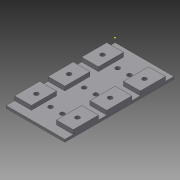
# Autodesk Inventor part: parking lot frame
Saved by Autodesk Inventor 2015 (Build 190159000, 159)
## iProperties
Created: 2015-10-07
Part Number: parking lot frame
Material: Generic
Document SubType Name: Modeling
Designer: Jason
Density: 1 g/cm^3
Appearance: Default
Author: Jason
Autodesk Inventor part; units mm, degrees
ref_plane "YZ Plane" through (0, 0, 0) normal (1, 0, 0) x (0, 1, 0)
ref_plane "XZ Plane" through (0, 0, 0) normal (0, 1, 0) x (-1, 0, 0)
ref_plane "XY Plane" through (0, 0, 0) normal (0, 0, 1) x (1, 0, 0)
sketch "Sketch1" plane through (0, 0, 0) normal (0, 0, 1) x (1, 0, 0)
  line L0 (0, 0) -> (70, 0)
  line L1 (70, 0) -> (70, -130)
  line L2 (70, -130) -> (0, -130)
  line L3 (0, -130) -> (0, 0)
  line L4 (0, -10) -> (20, -10)
  line L5 (20, -10) -> (20, -40)
  line L6 (20, -40) -> (0, -40)
  line L7 (0, -40) -> (0, -10)
  line L8 (50, -10) -> (70, -10)
  line L9 (70, -10) -> (70, -40)
  line L10 (70, -40) -> (50, -40)
  line L11 (50, -40) -> (50, -10)
  line L12 (0, -50) -> (20, -50)
  line L13 (20, -50) -> (20, -80)
  line L14 (20, -80) -> (0, -80)
  line L15 (0, -80) -> (0, -50)
  line L16 (50, -50) -> (70, -50)
  line L17 (70, -50) -> (70, -80)
  line L18 (70, -80) -> (50, -80)
  line L19 (50, -80) -> (50, -50)
  line L20 (0, -90) -> (20, -90)
  line L21 (20, -90) -> (20, -120)
  line L22 (20, -120) -> (0, -120)
  line L23 (0, -120) -> (0, -90)
  line L24 (50, -90) -> (70, -90)
  line L25 (70, -90) -> (70, -120)
  line L26 (70, -120) -> (50, -120)
  line L27 (50, -120) -> (50, -90)
  dimension "d0" = 70
  dimension "d1" = 130
  dimension "d2" = 20
  dimension "d3" = 30
  dimension "d4" = 20
  dimension "d5" = 30
  dimension "d6" = 20
  dimension "d7" = 30
  dimension "d8" = 20
  dimension "d9" = 30
  dimension "d10" = 20
  dimension "d11" = 30
  dimension "d12" = 20
  dimension "d13" = 30
  dimension "d14" = 10
  dimension "d15" = 10
  dimension "d16" = 10
  dimension "d17" = 10
  dimension "d18" = 10
  dimension "d19" = 0
  dimension "d20" = 30
  constraints: 56 end point, 14 parallel, 7 horizontal, 7 perpendicular, 5 point on line
  measures "d0" distance of L1.end L2.end
  measures "d1" distance between parallel lines of L2 L0
  measures "d2" distance of L5.end L6.end
  measures "d3" distance of L4.end L5.end
  measures "d4" distance of L9.end L10.end
  measures "d5" distance of L8.end L9.end
  measures "d6" distance of L13.end L14.end
  measures "d7" distance of L12.end L13.end
  measures "d8" distance of L17.end L18.end
  measures "d9" distance of L16.end L17.end
  measures "d10" distance of L21.end L22.end
  measures "d11" distance of L20.end L21.end
  measures "d12" distance of L25.end L26.end
  measures "d13" distance of L24.end L25.end
  measures "d14" distance between parallel lines of L0 L4
  measures "d15" distance between parallel lines of L12 L6
  measures "d16" distance between parallel lines of L20 L14
  measures "d17" distance between parallel lines of L16 L10
  measures "d18" distance between parallel lines of L24 L18
  measures "d19" distance between parallel lines of L23 L3
  measures "d20" distance between parallel lines of L27 L21
extrude "Extrusion1" add sketch "Sketch1" along normal blind 3 contours L0 L1 L8 L11 L10 L16 L19 L18 L24 L27 L26 L2 L3 L22 L21 L20 L14 L13 L12 L6 L5 L4
sketch "Sketch6" plane through (0, 0, 0) normal (0, 0, -1) x (-1, 0, 0)
  line L0 (-50, -10) -> (-70, -10)
  line L1 (-70, -10) -> (-70, -40)
  line L2 (-70, -40) -> (-50, -40)
  line L3 (-50, -40) -> (-50, -10)
  line L4 (-20, -10) -> (0, -10)
  line L5 (0, -10) -> (0, -40)
  line L6 (0, -40) -> (-20, -40)
  line L7 (-20, -40) -> (-20, -10)
  line L8 (-20, -50) -> (0, -50)
  line L9 (0, -50) -> (0, -80)
  line L10 (0, -80) -> (-20, -80)
  line L11 (-20, -80) -> (-20, -50)
  line L12 (0, -90) -> (-20, -90)
  line L13 (-20, -90) -> (-20, -120)
  line L14 (-20, -120) -> (0, -120)
  line L15 (0, -120) -> (0, -90)
  line L16 (-50, -90) -> (-70, -90)
  line L17 (-70, -90) -> (-70, -120)
  line L18 (-70, -120) -> (-50, -120)
  line L19 (-50, -120) -> (-50, -90)
  line L20 (-70, -80) -> (-50, -80)
  line L21 (-50, -80) -> (-50, -50)
  line L22 (-50, -50) -> (-70, -50)
  line L23 (-70, -50) -> (-70, -80)
  point P0 (0, 0)
  constraints: 48 end point, 12 parallel, 6 horizontal, 6 perpendicular
extrude "Extrusion3" add sketch "Sketch6" against normal blind 8
sketch "Sketch7" plane through (0, 0, 8) normal (0, 0, 1) x (1, 0, 0)
  point P0 (0, 0)
sketch "Sketch8" plane through (0, 0, 8) normal (0, 0, 1) x (1, 0, 0)
  circle A0 centre (10, -25) radius 2.6
  circle A1 centre (28, -25) radius 2.6
  circle A2 centre (42, -25) radius 2.6
  circle A3 centre (60, -25) radius 2.6
  circle A4 centre (10, -65) radius 2.6
  circle A5 centre (28, -65) radius 2.6
  circle A6 centre (42, -65) radius 2.6
  circle A7 centre (59, -65) radius 2.6
  circle A8 centre (11, -105) radius 2.6
  circle A9 centre (28, -105) radius 2.6
  circle A10 centre (42, -105) radius 2.6
  circle A11 centre (60, -105) radius 2.6
  line L0 (20, -10) -> (0, -10) projected
  line L1 (20, -40) -> (20, -10) projected
  line L2 (50, -10) -> (50, -40) projected
  line L3 (70, -10) -> (50, -10) projected
  line L4 (70, -40) -> (70, -10) projected
  line L5 (20, -50) -> (0, -50) projected
  line L6 (20, -90) -> (0, -90) projected
  line L7 (50, -50) -> (50, -80) projected
  point P0 (0, 0)
  dimension "d29" = 5.2
  dimension "d30" = 5.2
  dimension "d31" = 5.2
  dimension "d32" = 5.2
  dimension "d33" = 5.2
  dimension "d34" = 5.2
  dimension "d35" = 5.2
  dimension "d36" = 5.2
  dimension "d37" = 5.2
  dimension "d38" = 5.2
  dimension "d39" = 5.2
  dimension "d40" = 5.2
  dimension "d41" = 15
  dimension "d42" = 10
  dimension "d43" = 8
  dimension "d44" = 8
  dimension "d45" = 15
  dimension "d46" = 10
  dimension "d47" = 15
  dimension "d48" = 15
  dimension "d49" = 8
  constraints: 12 centre point
  measures "d29" diameter of A0
  measures "d30" diameter of A1
  measures "d31" diameter of A2
  measures "d32" diameter of A3
  measures "d33" diameter of A4
  measures "d34" diameter of A5
  measures "d35" diameter of A6
  measures "d36" diameter of A7
  measures "d37" diameter of A8
  measures "d38" diameter of A9
  measures "d39" diameter of A10
  measures "d40" diameter of A11
  measures "d41" distance from line of L0 A0.centre
  measures "d42" distance from line of L1 A0.centre
  measures "d43" distance from line of A1.centre L1
  measures "d44" distance from line of L2 A2.centre
  measures "d45" distance from line of L3 A3.centre
  measures "d46" distance from line of L4 A3.centre
  measures "d47" distance from line of L5 A4.centre
  measures "d48" distance from line of L6 A8.centre
  measures "d49" distance from line of L7 A6.centre
extrude "Extrusion4" cut sketch "Sketch8" against normal through all
body "Solid1"
